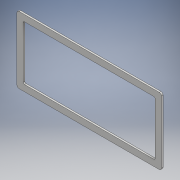
# Autodesk Inventor part: layer2
Saved by Autodesk Inventor 2017 (Build 210142000, 142)
## iProperties
Created: 2021-06-16
Part Number: layer2
Material: Generic
Document SubType Name: Modeling
Designer: Jack
Density: 1 g/cm^3
Appearance: Default
Author: Jack
Autodesk Inventor part; units mm, degrees
ref_plane "YZ Plane" through (0, 0, 0) normal (1, 0, 0) x (0, 1, 0)
ref_plane "XZ Plane" through (0, 0, 0) normal (0, 1, 0) x (-1, 0, 0)
ref_plane "XY Plane" through (0, 0, 0) normal (0, 0, 1) x (1, 0, 0)
sketch "Sketch1" plane through (0, 0, 0) normal (0, 1, 0) x (-1, 0, 0)
  line L0 (-163.5112, 73.4938) -> (-163.5112, -76.3312)
  line L1 (-158.5112, 78.4938) -> (177.0518, 78.4938)
  arc A0 (-158.5112, 78.4938) -> (-163.5112, 73.4938) centre (-158.5112, 73.4938) ccw
  arc A1 (-163.5112, -76.3312) -> (-158.5112, -81.3312) centre (-158.5112, -76.3312) ccw
  line L2 (182.0518, -76.3312) -> (182.0518, 73.4938)
  line L3 (177.0518, -81.3312) -> (-158.5112, -81.3312)
  arc A2 (177.0518, -81.3312) -> (182.0518, -76.3312) centre (177.0518, -76.3312) ccw
  arc A3 (182.0518, 73.4938) -> (177.0518, 78.4938) centre (177.0518, 73.4938) ccw
  line L4 (-145.5232, 63.4943) -> (164.0397, 63.4943)
  line L5 (-148.5112, 60.4941) -> (-148.5112, -63.3312)
  line L6 (167.0517, 60.4941) -> (167.0517, -63.3312)
  line L7 (-145.5112, -66.3312) -> (164.0517, -66.3312)
  arc A4 (-145.5112, 63.4943) -> (-148.5112, 60.4648) centre (-145.5112, 60.4941) ccw
  arc A5 (167.0517, 60.4941) -> (164.0397, 63.4943) centre (164.1459, 60.5889) ccw
  arc A6 (164.0517, -66.3312) -> (167.0517, -63.3312) centre (164.0517, -63.3312) ccw
  arc A7 (-148.5112, -63.3312) -> (-145.5112, -66.3312) centre (-145.5112, -63.3312) ccw
  point P0 (0, 0)
  constraints: 16 end point, 16 point on circle, 8 centre point, 2 point on line
extrude "Extrusion1" add sketch "Sketch1" along normal blind 4
body "Solid1"
